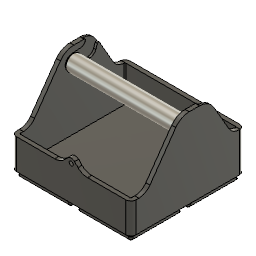
SnapTools-2U-Solder-Wire-Holder (Autodesk Fusion 360 design; units mm, degrees)
Autodesk Fusion 360 part; units mm, degrees
sketch "Sketch1" plane through (0, 0, 0) normal (0, 1, 0) x (1, 0, 0) in component "SnapTools-2U-Solder-Wire-Holder-Base"
  line L0 (-41.75, -2.4) -> (-2.4, -2.4)
  line L1 (-2.4, -2.4) -> (-2.4, -39.6)
  line L2 (-2.4, -39.6) -> (-41.75, -39.6)
  line L3 (-41.75, -39.6) -> (-41.75, -2.4)
  line L4 (-41.75, 2.4) -> (-2.4, 2.4)
  line L5 (-2.4, 2.4) -> (-2.4, 39.6)
  line L6 (-2.4, 39.6) -> (-41.75, 39.6)
  line L7 (-41.75, 39.6) -> (-41.75, 2.4)
  line L8 (-41.75, 2.4) -> (-2.4, 39.6) construction
  circle A0 centre (-35.8263, 8) radius 3.125
  line L9 (-22.075, 21) -> (-2.4, 21) construction
  line L10 (-2.4, 2.4) -> (-22.075, 21) construction
  circle A1 centre (-8.3237, 8) radius 3.125
  circle A2 centre (-8.3237, 34) radius 3.125
  circle A3 centre (-35.8263, 34) radius 3.125
  line L11 (0, 0) -> (34, 0) construction
  circle A4 centre (-35.8263, -34) radius 3.125
  circle A5 centre (-35.8263, -8) radius 3.125
  circle A6 centre (-8.3237, -8) radius 3.125
  circle A7 centre (-8.3237, -34) radius 3.125
  circle A8 centre (-22.075, 21) radius 5.125
  circle A9 centre (-22.075, -21) radius 5.125
  line L12 (0, 0) -> (0, 26) construction
  line L13 (2.4, 2.4) -> (2.4, 39.6)
  line L14 (41.75, 2.4) -> (2.4, 2.4)
  line L15 (41.75, 39.6) -> (41.75, 2.4)
  line L16 (2.4, 39.6) -> (41.75, 39.6)
  circle A10 centre (35.8263, 34) radius 3.125
  circle A11 centre (22.075, 21) radius 5.125
  circle A12 centre (8.3237, 34) radius 3.125
  circle A13 centre (8.3237, 8) radius 3.125
  circle A14 centre (35.8263, 8) radius 3.125
  circle A15 centre (35.8263, -8) radius 3.125
  circle A16 centre (8.3237, -8) radius 3.125
  line L17 (2.4, -39.6) -> (41.75, -39.6)
  line L18 (41.75, -39.6) -> (41.75, -2.4)
  line L19 (2.4, -2.4) -> (2.4, -39.6)
  line L20 (41.75, -2.4) -> (2.4, -2.4)
  circle A17 centre (22.075, -21) radius 5.125
  circle A18 centre (8.3237, -34) radius 3.125
  circle A19 centre (35.8263, -34) radius 3.125
  dimension "d15" = 39.35
  dimension "d16" = 4.8
  dimension "d18" = 2.4
  dimension "d19" = 79.2
  dimension "d20" = 39.6
  dimension "d21" = 37.2
  dimension "d25" = 5.6
  dimension "d26" = 6.25
  dimension "d27" = 6.25
  dimension "d28" = 5.6
  dimension "d110" = 10.25
  constraint horizontal L0
  constraint vertical L1
  constraint horizontal L2
  constraint vertical L3
  constraint horizontal L4
  constraint vertical L5
  constraint horizontal L6
  constraint vertical L7
  constraint collinear L1 L5
  constraint collinear L3 L7
  constraint coincident L8 A0.centre
  constraint midpoint L8 L9.start
  constraint midpoint L5 L9.end
  constraint coincident L10 A1.centre
  constraint symmetric A0 L9 A3
  constraint symmetric L9 A1 A2
  constraint coincident L11.start L12.start
  constraint parallel L4 L11
  constraint symmetric A0 L11 A5
  constraint symmetric A1 L11 A6
  constraint symmetric A2 L11 A7
  constraint symmetric A3 L11 A4
  constraint coincident L9.start L10.end
  constraint symmetric L11 A8 A9
  constraint perpendicular L11 L12
  constraint symmetric L0.start L12 L18.end
  constraint symmetric L0.end L12 L19.start
  constraint symmetric L1.end L12 L17.start
  constraint symmetric L2.end L12 L17.end
  constraint symmetric L4.start L12 L14.start
  constraint symmetric L4.end L12 L13.start
  constraint symmetric L5.end L12 L13.end
  constraint symmetric L6.end L12 L15.start
  constraint symmetric A0 L12 A14
  constraint symmetric A1 L12 A13
  constraint symmetric A2 L12 A12
  constraint symmetric A3 L12 A10
  constraint symmetric A4 L12 A19
  constraint symmetric A5 L12 A15
  constraint symmetric A6 L12 A16
  constraint symmetric A7 L12 A18
  constraint symmetric A8 L12 A11
  constraint symmetric A9 L12 A17
  measures "d15" distance of L1.end L2.end
  measures "d16" distance of L0 L4
  measures "d18" vertical distance of L11.start L0.end
  measures "d19" distance of L2 L6
  measures "d20" distance of L11.start L2
  measures "d21" distance of L0 L2
  measures "d25" distance of L4 A0.centre
  measures "d26" diameter of A0
  measures "d27" diameter of A1
  measures "d28" distance of L4 A1.centre
  measures "d74" angle of L4.start
  measures "d110" diameter of A8
extrude "Extrude1" add sketch "Sketch1" along normal blind 2.6 contours L0 L1 L2 L3 | L4 L5 L6 L7 | A0 | A1 | A2 | A3 | A4 | A5 | A6 | A7 | A8 | A9 | L13 L14 L15 L16 | A10 | A11 | A12 | A13 | A14 | A15 | A16 | L17 L18 L19 L20 | A17 | A18 | A19 makes body 1 at (-28.6333, 0, 27.2) makes body 2 at (-15.5167, 0, -27.2) makes body 3 at (15.5167, 0, 14.8) makes body 4 at (15.5167, 0, -27.2) in component "SnapTools-2U-Solder-Wire-Holder-Base"
fillet "Fillet3" radius 1.6 16 edges at (-2.4, 1.3, 2.4) (-41.75, 1.3, 2.4) (-41.75, 1.3, 39.6) (-2.4, 1.3, 39.6) (-41.75, 1.3, -39.6) (-41.75, 1.3, -2.4) (-2.4, 1.3, -2.4) (-2.4, 1.3, -39.6) (2.4, 1.3, 39.6) (2.4, 1.3, 2.4) (41.75, 1.3, 39.6) (41.75, 1.3, 2.4) (41.75, 1.3, -2.4) (2.4, 1.3, -2.4) (2.4, 1.3, -39.6) (41.75, 1.3, -39.6) on bodies 1 2 3 4 in component "SnapTools-2U-Solder-Wire-Holder-Base"
chamfer "Chamfer4" distance 0.8 angle 45 32 edges at (-41.75, 0, -21) (-41.2814, 0, -2.8686) (-22.075, 0, -2.4) (-2.8686, 0, -2.8686) (-2.4, 0, -21) (-2.8686, 0, -39.1314) (-22.075, 0, -39.6) (-41.2814, 0, -39.1314) (-41.75, 0, 21) (-41.2814, 0, 2.8686) (-22.075, 0, 2.4) (-2.8686, 0, 2.8686) (-2.4, 0, 21) (-2.8686, 0, 39.1314) (-22.075, 0, 39.6) (-41.2814, 0, 39.1314) (22.075, 0, 39.6) (41.2814, 0, 39.1314) (41.75, 0, 21) (41.2814, 0, 2.8686) (22.075, 0, 2.4) (2.8686, 0, 2.8686) (2.4, 0, 21) (2.8686, 0, 39.1314) (22.075, 0, -2.4) (2.8686, 0, -2.8686) (2.4, 0, -21) (2.8686, 0, -39.1314) (22.075, 0, -39.6) (41.2814, 0, -39.1314) (41.75, 0, -21) (41.2814, 0, -2.8686) on bodies 1 2 3 4 in component "SnapTools-2U-Solder-Wire-Holder-Base"
extrude "Extrude7" add 4 faces at (-16.05, 2.6, -27.2) (16.05, 2.6, -27.2) (16.05, 2.6, 14.8) (-28.1, 2.6, 27.2) along direction (0, 1, 0) blind 2.15 draft 45 on bodies 1 2 3 4 bodies 2 3 1 4 in component "SnapTools-2U-Solder-Wire-Holder-Base"
sketch "Sketch6" plane through (0, 4.75, 0) normal (0, 1, 0) x (-1, 0, 0) in component "SnapTools-2U-Solder-Wire-Holder-Base"
  line L0 (0.25, -4) -> (0.25, -38)
  arc A0 (0.25, -38) -> (4, -41.75) centre (4, -38) ccw
  line L1 (4, -41.75) -> (40.15, -41.75)
  arc A1 (40.15, -41.75) -> (43.9, -38) centre (40.15, -38) ccw
  line L2 (43.9, -38) -> (43.9, -4)
  arc A2 (43.9, -4) -> (40.15, -0.25) centre (40.15, -4) ccw
  line L3 (40.15, -0.25) -> (4, -0.25)
  arc A3 (4, -0.25) -> (0.25, -4) centre (4, -4) ccw
  line L4 (40.15, 41.75) -> (4, 41.75)
  arc A4 (4, 41.75) -> (0.25, 38) centre (4, 38) ccw
  line L5 (0.25, 38) -> (0.25, 4)
  arc A5 (0.25, 4) -> (4, 0.25) centre (4, 4) ccw
  line L6 (4, 0.25) -> (40.15, 0.25) construction
  arc A6 (40.15, 0.25) -> (43.9, 4) centre (40.15, 4) ccw
  line L7 (43.9, 4) -> (43.9, 38)
  arc A7 (43.9, 38) -> (40.15, 41.75) centre (40.15, 38) ccw
  line L8 (43.9, -4) -> (43.9, 4)
  line L9 (40.15, 41.75) -> (4, 41.75)
  arc A8 (4, 41.75) -> (0.25, 38) centre (4, 38) ccw
  line L10 (0.25, 38) -> (0.25, 4)
  arc A9 (0.25, 4) -> (4, 0.25) centre (4, 4) ccw
  line L11 (4, 0.25) -> (40.15, 0.25)
  arc A10 (40.15, 0.25) -> (43.9, 4) centre (40.15, 4) ccw
  line L12 (43.9, 4) -> (43.9, 38)
  arc A11 (43.9, 38) -> (40.15, 41.75) centre (40.15, 38) ccw
  line L13 (-43.9, 38) -> (-43.9, 4)
  arc A12 (-43.9, 4) -> (-40.15, 0.25) centre (-40.15, 4) ccw
  line L14 (-40.15, 0.25) -> (-4, 0.25)
  arc A13 (-4, 0.25) -> (-0.25, 4) centre (-4, 4) ccw
  line L15 (-0.25, 4) -> (-0.25, 38)
  arc A14 (-0.25, 38) -> (-4, 41.75) centre (-4, 38) ccw
  line L16 (-4, 41.75) -> (-40.15, 41.75)
  arc A15 (-40.15, 41.75) -> (-43.9, 38) centre (-40.15, 38) ccw
  line L17 (-43.9, -4) -> (-43.9, -38)
  arc A16 (-43.9, -38) -> (-40.15, -41.75) centre (-40.15, -38) ccw
  line L18 (-40.15, -41.75) -> (-4, -41.75)
  arc A17 (-4, -41.75) -> (-0.25, -38) centre (-4, -38) ccw
  line L19 (-0.25, -38) -> (-0.25, -4)
  arc A18 (-0.25, -4) -> (-4, -0.25) centre (-4, -4) ccw
  line L20 (-4, -0.25) -> (-40.15, -0.25)
  arc A19 (-40.15, -0.25) -> (-43.9, -4) centre (-40.15, -4) ccw
  line L21 (0.25, -4) -> (0.25, -38)
  arc A20 (0.25, -38) -> (4, -41.75) centre (4, -38) ccw
  line L22 (4, -41.75) -> (40.15, -41.75)
  arc A21 (40.15, -41.75) -> (43.9, -38) centre (40.15, -38) ccw
  line L23 (43.9, -38) -> (43.9, -4)
  arc A22 (43.9, -4) -> (40.15, -0.25) centre (40.15, -4) ccw
  line L24 (40.15, -0.25) -> (4, -0.25)
  arc A23 (4, -0.25) -> (0.25, -4) centre (4, -4) ccw
  line L25 (4, 41.75) -> (-4, 41.75)
  line L26 (-43.9, 4) -> (-43.9, -4)
  line L27 (-4, -41.75) -> (4, -41.75)
  constraint coincident L2.end A2.start
  constraint coincident A6.end L7.start
  constraint coincident L4.end A4.start
  constraint coincident A14.end L16.start
  constraint coincident L13.end A12.start
  constraint coincident L17.start A19.end
  constraint coincident L18.end A17.start
  constraint coincident A0.end L1.start
extrude "Extrude10" add sketch "Sketch6" along normal blind 2.25 bodies 1 3 4 2 in component "SnapTools-2U-Solder-Wire-Holder-Base"
extrude "Extrude5" cut sketch "Sketch1" along normal blind 2 contours A0 | A1 | A2 | A3 | A4 | A5 | A6 | A7 | A10 | A12 | A13 | A14 | A15 | A16 | A18 | A19 bodies 1 in component "SnapTools-2U-Solder-Wire-Holder-Base"
extrude "Extrude6" cut 16 faces at (-35.0627, 2, -35.019) (-7.3389, 2, -33.241) (-36.6468, 2, -8.8534) (-7.9632, 2, -7.548) (-7.4113, 2, 8.7544) (-36.8217, 2, 6.89) (-35.0627, 2, 32.981) (-7.3389, 2, 34.759) (9.0194, 2, 36.0626) (36.5899, 2, 32.981) (9.236, 2, 8.7544) (34.831, 2, 6.89) (34.831, 2, -9.11) (7.9948, 2, -9.1373) (8.9223, 2, -35.9409) (36.5899, 2, -35.019) along direction (0, 1, 0) blind 5 draft -55 on bodies 1 bodies 1 in component "SnapTools-2U-Solder-Wire-Holder-Base"
sketch "Sketch1 (2)" plane through (0, 7, 0) normal (0, 1, 0) x (-1, 0, 0) in component "SnapTools-2U-Solder-Wire-Holder-Base"
  line L0 (-40.15, -41.75) -> (40.15, -41.75)
  arc A0 (40.15, -41.75) -> (43.9, -38) centre (40.15, -38) ccw
  line L1 (43.9, -38) -> (43.9, 38)
  line L2 (31.464, -31.8398) -> (-31.536, -31.8398) construction
  line L3 (-31.536, -31.8398) -> (-31.536, 31.1602) construction
  line L4 (-31.536, 31.1602) -> (31.464, 31.1602) construction
  line L5 (31.464, 31.1602) -> (31.464, -31.8398) construction
  arc A1 (43.9, 38) -> (40.15, 41.75) centre (40.15, 38) ccw
  line L6 (40.15, 41.75) -> (-40.15, 41.75)
  arc A2 (-40.15, 41.75) -> (-43.9, 38) centre (-40.15, 38) ccw
  line L7 (-43.9, 38) -> (-43.9, -38)
  arc A3 (-43.9, -38) -> (-40.15, -41.75) centre (-40.15, -38) ccw
  line L8 (-40.15, -38.75) -> (40.15, -38.75)
  arc A4 (40.15, -38.75) -> (40.9, -38) centre (40.15, -38) ccw
  line L9 (40.9, -38) -> (40.9, 38)
  arc A5 (40.9, 38) -> (40.15, 38.75) centre (40.15, 38) ccw
  line L10 (40.15, 38.75) -> (-40.15, 38.75)
  arc A6 (-40.15, 38.75) -> (-40.9, 38) centre (-40.15, 38) ccw
  line L11 (-40.9, 38) -> (-40.9, -38)
  arc A7 (-40.9, -38) -> (-40.15, -38.75) centre (-40.15, -38) ccw
  dimension "d67" = 63
  dimension "d68" = 63
  constraint horizontal L2
  constraint vertical L3
  constraint horizontal L4
  constraint vertical L5
  measures "d67" distance of L2.start L2.end
  measures "d68" distance of L2.start L4.end
extrude "Extrude11" add sketch "Sketch1 (2)" along normal blind 56.5 bodies 1 in component "SnapTools-2U-Solder-Wire-Holder-Base"
sketch "Sketch2" plane through (-43.9, 0, 0) normal (-1, 0, 0) x (0, 0, 1) in component "SnapTools-2U-Solder-Wire-Holder-Base"
  line L0 (-38, 4.75) -> (-4, 4.75)
  line L1 (38, 63.5) -> (-38, 63.5)
  line L2 (-38, 63.5) -> (-38, 4.75)
  line L3 (-38, 7) -> (-38.75, 7)
  line L4 (-38, 7) -> (38, 7)
  circle A0 centre (0, 53.5) radius 5 construction
  circle A1 centre (0, 53.5) radius 31.5 construction
  line L5 (41.75, 4.75) -> (41.75, 63.5)
  line L6 (41.75, 27) -> (30.7632, 27)
  line L7 (30.7632, 27) -> (5.2057, 63.5)
  line L8 (-15.5885, 63.5) -> (-32.909, 33.5)
  line L9 (-41.75, 4.75) -> (-41.75, 63.5)
  line L10 (-32.909, 33.5) -> (-41.75, 33.5)
  line L11 (0, 7) -> (0, 63.5) construction
  line L12 (-15.5885, 63.5) -> (-41.75, 63.5)
  line L13 (5.2057, 63.5) -> (41.75, 63.5)
  line L14 (-4, 4.75) -> (4, 4.75)
  line L15 (4, 4.75) -> (38, 4.75)
  line L16 (38, 4.75) -> (38, 63.5)
  line L17 (38.75, 7) -> (38, 7)
  line L18 (38.75, 7) -> (38, 7)
  line L19 (38, 7) -> (-38, 7)
  line L20 (-38, 7) -> (-38.75, 7)
  dimension "d71" = 10
  dimension "d73" = 63
  dimension "d74" = 125
  dimension "d75" = 10
  dimension "d76" = 120
  dimension "d77" = 30
  dimension "d78" = 18.5
  dimension "d130" = 46.5
  dimension "d132" = 20
  constraint concentric A0 A1
  constraint coincident L5 L6.start
  constraint coincident L1 L7.end
  constraint coincident L1 L8.start
  constraint coincident L9 L10.end
  constraint perpendicular L9 L10
  constraint midpoint L1 L11.end
  constraint coincident A0.centre L11
  constraint coincident L9.end L12.end
  constraint coincident L5.end L13.end
  constraint midpoint L4 L11.start
  constraint perpendicular L5 L6
  measures "d71" diameter of A0
  measures "d73" diameter of A1
  measures "d74" angle of L6 L7
  measures "d75" distance of A0.centre L7
  measures "d76" angle of L8 L10
  measures "d77" distance of L1 L10
  measures "d78" distance of A0.centre L8
  measures "d130" distance of A0.centre L19
  measures "d132" distance of L4 L6
extrude "Extrude12" cut sketch "Sketch2" against normal through all contours L2 L9 L10 L12 | L1 L2 L8 L10 L12 | L5 L6 L13 L16 | L1 L6 L7 L13 L16 bodies 1 in component "SnapTools-2U-Solder-Wire-Holder-Base"
sketch "Sketch3" plane through (40.9, 0, 0) normal (-1, 0, 0) x (0, 0, 1) in component "SnapTools-2U-Solder-Wire-Holder-Base"
  line L0 (0, 0) -> (0, 69) construction
  circle A0 centre (0, 53.5) radius 5 construction
  circle A1 centre (0, 53.5) radius 5.25
  line L1 (0.4576, 58.73) -> (-6.6468, 59.3516)
  line L2 (-9.2044, 61.3141) -> (-10, 63.5)
  line L3 (-0.4576, 48.27) -> (-12.9564, 49.3635)
  line L4 (-17.2191, 52.6344) -> (-19.0142, 57.5664)
  arc A2 (-9.2044, 61.3141) -> (-6.6468, 59.3516) centre (-6.3853, 62.3402) ccw
  arc A3 (-17.2191, 52.6344) -> (-12.9564, 49.3635) centre (-12.5206, 54.3445) ccw
  line L5 (-32.909, 33.5) -> (-38, 33.5)
  line L6 (-38, 33.5) -> (-38, 7)
  line L7 (-38, 7) -> (38, 7)
  line L8 (38, 7) -> (38, 27)
  line L9 (38, 27) -> (30.7632, 27)
  line L10 (30.7632, 27) -> (5.2057, 63.5)
  line L11 (5.2057, 63.5) -> (-15.5885, 63.5)
  line L12 (-15.5885, 63.5) -> (-32.909, 33.5)
  dimension "d80" = 10
  dimension "d82" = 0.25
  dimension "d83" = 10.5
  dimension "d86" = 3
  dimension "d87" = 5
  dimension "d88" = 10
  dimension "d133" = 46.5
  dimension "d134" = 70
  dimension "d135" = 5
  constraint coincident L0 A0.centre
  constraint coincident A1 L1.start
  constraint coincident A1 L3.start
  constraint parallel L2 L4
  constraint tangent A1 L1
  constraint tangent A1 L3
  constraint parallel L1 L3
  constraint tangent L2 A2
  constraint tangent L1 A2
  constraint tangent L4 A3
  constraint tangent L3 A3
  constraint coincident L4.end L12
  constraint coincident L2.end L11
  constraint coincident L0.start origin
  constraint vertical L0
  measures "d80" diameter of A0
  measures "d83" distance of L2 L4
  measures "d86" radius of A2
  measures "d87" radius of A3
  measures "d88" horizontal distance of A0.centre L2.end
  measures "d133" distance of A0.centre L7
  measures "d134" angle of L2 L11
  measures "d135" angle of L1 L11
extrude "Extrude13" cut sketch "Sketch3" against normal blind 1.6 contours A1 | A1 L1 L2 L3 L4 A2 A3 L11 L12 bodies 1 in component "SnapTools-2U-Solder-Wire-Holder-Base"
extrude "Extrude14" cut 1 faces at (42.5, 52.3283, -6.6869) along direction (-1, 0, 0) blind 1.6 from surface at 83.4 on bodies 1 bodies 1 in component "SnapTools-2U-Solder-Wire-Holder-Base"
sketch "Sketch7" plane through (0, 0, 41.75) normal (0, 0, 1) x (1, 0, 0) in component "SnapTools-2U-Solder-Wire-Holder-Base"
  line L0 (40.15, 27) -> (-40.15, 27)
  line L1 (-40.15, 27) -> (-40.15, 4.75)
  circle A0 centre (0, 30) radius 1.5
  circle A1 centre (0, 30) radius 3.5
  line L2 (0, 27) -> (0, 36.6034) construction
  line L3 (-2.4749, 32.4749) -> (-7.9497, 27)
  line L4 (2.4749, 32.4749) -> (7.9497, 27)
  line L5 (-40.15, 4.75) -> (-4, 4.75)
  line L6 (-4, 4.75) -> (4, 4.75)
  line L7 (4, 4.75) -> (40.15, 4.75)
  line L8 (40.15, 4.75) -> (40.15, 27)
  dimension "d95" = 3
  dimension "d96" = 2
  dimension "d97" = 3
  dimension "d98" = 45
  dimension "d99" = 45
  constraint midpoint L0 L2.start
  constraint perpendicular L0 L2
  constraint coincident A0.centre L2
  constraint coincident A1 L3.start
  constraint coincident L0 L3.end
  constraint coincident A1 L4.start
  constraint coincident L0 L4.end
  constraint tangent A1 L4
  constraint tangent A1 L3
  measures "d95" diameter of A0
  measures "d97" distance of A0.centre L2.start
  measures "d98" angle of L0 L3
  measures "d99" angle of L0 L4
extrude "Extrude15" add sketch "Sketch7" against normal up to surface (3 mm away) contours L0 A1 L4 | L0 A1 | L0 A1 L3 picked at (-0.0374, 27.5014) bodies 1 in component "SnapTools-2U-Solder-Wire-Holder-Base"
fillet "Fillet4" radius 10 2 edges at (-7.9497, 27, 40.25) (7.9497, 27, 40.25) on bodies 1 in component "SnapTools-2U-Solder-Wire-Holder-Base"
fillet "Fillet5" radius 12 4 edges at (42.4, 63.5, 5.2057) (-42.4, 63.5, 5.2057) (-43.2, 63.5, -15.5885) (43.2, 63.5, -15.5885) on bodies 1 in component "SnapTools-2U-Solder-Wire-Holder-Base"
fillet "Fillet7" radius 10 4 edges at (-42.4, 27, 30.7632) (42.4, 27, 30.7632) (42.4, 33.5, -32.909) (-42.4, 33.5, -32.909) on bodies 1 in component "SnapTools-2U-Solder-Wire-Holder-Base"
fillet "Fillet6" radius 0.8 4 edges at (-41.7, 57.5661, -19.0141) (41.7, 57.5661, -19.0141) (41.7, 63.4279, -9.9738) (-41.7, 63.4279, -9.9738) on bodies 1 in component "SnapTools-2U-Solder-Wire-Holder-Base"
extrude "Extrude16" cut sketch "Sketch1" along normal blind 5.25 contours A8 | A9 | A11 | A17 bodies 1 in component "SnapTools-2U-Solder-Wire-Holder-Base"
extrude "Extrude17" cut 4 faces at (-20.7203, 5.25, -21.7134) (-20.7203, 5.25, 20.2866) (23.4297, 5.25, -21.7134) (23.4297, 5.25, 20.2866) along direction (0, 1, 0) blind 0.8 draft -60 on bodies 1 bodies 1 in component "SnapTools-2U-Solder-Wire-Holder-Base"
sketch "Sketch1 (3)" plane through (42.5, 0, 0) normal (-1, 0, 0) x (0, 0, 1) in component "SnapTools-2U-Solder-Wire-Holder-Axle 10mm"
  line L0 (-18.4274, 55.9543) -> (-17.2191, 52.6344)
  arc A0 (-17.2191, 52.6344) -> (-12.9564, 49.3635) centre (-12.5206, 54.3445) ccw
  line L1 (-12.9564, 49.3635) -> (-0.4576, 48.27)
  line L2 (0.4576, 58.73) -> (-6.6468, 59.3516)
  arc A1 (-9.2044, 61.3141) -> (-6.6468, 59.3516) centre (-6.3853, 62.3402) ccw
  circle A2 centre (0, 53.5) radius 5
  line L3 (-9.2044, 61.3141) -> (-9.6086, 62.4247)
  arc A3 (-8.8709, 63.4982) -> (-19.0526, 57.5) centre (-8.6603, 51.5) ccw
  line L4 (-19.0526, 57.5) -> (-19.872, 56.0807)
  arc A4 (-18.4274, 55.9543) -> (-19.872, 56.0807) centre (-19.1792, 55.6807) ccw
  arc A5 (-0.4576, 48.27) -> (0.4576, 58.73) centre (0, 53.5) ccw
  arc A6 (-8.8709, 63.4982) -> (-9.6086, 62.4247) centre (-8.8569, 62.6983) ccw
  dimension "d115" = 10
  constraint coincident A2.centre A5.centre
  measures "d115" diameter of A2
extrude "Extrude1'" add sketch "Sketch1 (3)" along normal up to surface (85 mm away) separate body contours A2 makes body 5 in component "SnapTools-2U-Solder-Wire-Holder-Axle 10mm"
sketch "Sketch1 (4)" plane through (42.5, 0, 0) normal (-1, 0, 0) x (0, 0, 1) in component "SnapTools-2U-Solder-Wire-Holder-Axle 20mm"
  line L0 (-18.4274, 55.9543) -> (-17.2191, 52.6344)
  arc A0 (-17.2191, 52.6344) -> (-12.9564, 49.3635) centre (-12.5206, 54.3445) ccw
  line L1 (-12.9564, 49.3635) -> (-0.4576, 48.27)
  line L2 (0.4576, 58.73) -> (-6.6468, 59.3516)
  arc A1 (-9.2044, 61.3141) -> (-6.6468, 59.3516) centre (-6.3853, 62.3402) ccw
  circle A2 centre (0, 53.5) radius 5
  circle A3 centre (0, 53.5) radius 10
  line L3 (-9.2044, 61.3141) -> (-9.6086, 62.4247)
  arc A4 (-8.8709, 63.4982) -> (-19.0526, 57.5) centre (-8.6603, 51.5) ccw
  line L4 (-19.0526, 57.5) -> (-19.872, 56.0807)
  arc A5 (-18.4274, 55.9543) -> (-19.872, 56.0807) centre (-19.1792, 55.6807) ccw
  arc A6 (-0.4576, 48.27) -> (0.4576, 58.73) centre (0, 53.5) ccw
  arc A7 (-8.8709, 63.4982) -> (-9.6086, 62.4247) centre (-8.8569, 62.6983) ccw
  dimension "d115_1" = 10
  dimension "d119" = 20
  constraint concentric A2 A3
  constraint coincident A2.centre A3.centre
  measures "d115_1" diameter of A2
  measures "d119" diameter of A3
extrude "Extrude1''" add sketch "Sketch1 (4)" along normal up to surface (85 mm away) separate body contours A2 makes body 6 in component "SnapTools-2U-Solder-Wire-Holder-Axle 20mm"
extrude "Extrude2" add sketch "Sketch1 (4)" along normal up to surface (81.3 mm away) from surface at 1.85 contours L1 L2 A1 A3 A6 | L1 L2 A1 A3 A6 bodies 6 in component "SnapTools-2U-Solder-Wire-Holder-Axle 20mm"
chamfer "Chamfer1" distance 5 angle 45 2 edges at (-40.65, 49.8838, -9.3233) (40.65, 57.1162, -9.3233) on bodies 6 in component "SnapTools-2U-Solder-Wire-Holder-Axle 20mm"
sketch "Sketch1 (5)" plane through (42.5, 0, 0) normal (-1, 0, 0) x (0, 0, 1) in component "SnapTools-2U-Solder-Wire-Holder-Axle Parametric"
  line L0 (-18.4274, 55.9543) -> (-17.2191, 52.6344)
  arc A0 (-17.2191, 52.6344) -> (-12.9564, 49.3635) centre (-12.5206, 54.3445) ccw
  line L1 (-12.9564, 49.3635) -> (-0.4576, 48.27)
  line L2 (0.4576, 58.73) -> (-6.6468, 59.3516)
  arc A1 (-9.2044, 61.3141) -> (-6.6468, 59.3516) centre (-6.3853, 62.3402) ccw
  circle A2 centre (0, 53.5) radius 5
  circle A3 centre (0, 53.5) radius 5.75
  line L3 (-9.2044, 61.3141) -> (-9.6086, 62.4247)
  arc A4 (-8.8709, 63.4982) -> (-19.0526, 57.5) centre (-8.6603, 51.5) ccw
  line L4 (-19.0526, 57.5) -> (-19.872, 56.0807)
  arc A5 (-18.4274, 55.9543) -> (-19.872, 56.0807) centre (-19.1792, 55.6807) ccw
  arc A6 (-0.4576, 48.27) -> (0.4576, 58.73) centre (0, 53.5) ccw
  arc A7 (-8.8709, 63.4982) -> (-9.6086, 62.4247) centre (-8.8569, 62.6983) ccw
  dimension "d115_1_1" = 10
  dimension "d119_1" = 11.5
  constraint concentric A2 A3
  constraint coincident A2.centre A3.centre
  measures "d115_1_1" diameter of A2
  measures "d119_1" diameter of A3
extrude "Extrude1'''" add sketch "Sketch1 (5)" along normal up to surface (85 mm away) separate body contours A2 makes body 7 in component "SnapTools-2U-Solder-Wire-Holder-Axle Parametric"
extrude "Extrude2'" add sketch "Sketch1 (5)" along normal up to surface (81.3 mm away) from surface at 1.85 contours L1 L2 A3 A6 | L1 L2 A3 A6 bodies 7 in component "SnapTools-2U-Solder-Wire-Holder-Axle Parametric"
chamfer "Chamfer1'" distance 0.75 angle 45 2 edges at (-40.65, 51.4207, -5.3609) (40.65, 55.5793, -5.3609) on bodies 7 in component "SnapTools-2U-Solder-Wire-Holder-Axle Parametric"
sketch "Sketch4" plane through (40.9, 0, 0) normal (-1, 0, 0) x (0, 0, 1)
  arc A0 (-18.6485, 57) -> (-27.841, 52.7135) centre (-18.6485, 45) ccw
  line L0 (-27.841, 52.7135) -> (-29.0383, 51.2865)
  arc A1 (-36.4, 47.1405) -> (-29.0383, 51.2865) centre (-38.2309, 59) ccw
  line L1 (-36.4, 47.1405) -> (-36.4, 4.75)
  line L2 (-36.4, 4.75) -> (-5.6, 4.75)
  line L3 (-5.6, 4.75) -> (5.6, 4.75)
  line L4 (5.6, 4.75) -> (36.4, 4.75)
  line L5 (36.4, 4.75) -> (36.4, 22.8096)
  arc A2 (30.0399, 26.7571) -> (36.4, 22.8096) centre (39.2324, 34.4706) ccw
  line L6 (30.0399, 26.7571) -> (8.2599, 52.7135)
  arc A3 (8.2599, 52.7135) -> (-0.9326, 57) centre (-0.9326, 45) ccw
  line L7 (-0.9326, 57) -> (-18.6485, 57)
  circle A4 centre (-0.3007, 53.6477) radius 25
  circle A5 centre (-0.3007, 53.6477) radius 5
  line L8 (-4, 4.75) -> (-38, 4.75)
  line L9 (-38, 4.75) -> (-38, 42.0565)
  arc A6 (-20.7187, 55.7495) -> (-24.5775, 52.7135) centre (-15.385, 45) ccw
  line L10 (-20.7187, 55.7495) -> (-17.2191, 46.1344)
  arc A7 (-17.2191, 46.1344) -> (-12.9564, 42.8635) centre (-12.5207, 47.8445) ccw
  line L11 (-12.9564, 42.8635) -> (-4, 42.0799)
  line L12 (-4, 42.0799) -> (-4, 4.75)
  arc A8 (-38, 42.0565) -> (-29.9703, 46.2865) centre (-39.1629, 54) ccw
  line L13 (-29.9703, 46.2865) -> (-24.5775, 52.7135)
  arc A9 (-8.8709, 63.4982) -> (-9.6086, 62.4247) centre (-8.8569, 62.6983) ccw
  line L14 (-9.6086, 62.4247) -> (-9.2044, 61.3141)
  arc A10 (-9.2044, 61.3141) -> (-6.6468, 59.3516) centre (-6.3853, 62.3402) ccw
  line L15 (-6.6468, 59.3516) -> (0.4576, 58.73)
  arc A11 (-0.4576, 48.27) -> (0.4576, 58.73) centre (0, 53.5) ccw
  line L16 (-0.4576, 48.27) -> (-12.9564, 49.3635)
  arc A12 (-17.2191, 52.6344) -> (-12.9564, 49.3635) centre (-12.5206, 54.3445) ccw
  line L17 (-17.2191, 52.6344) -> (-18.4274, 55.9543)
  arc A13 (-18.4274, 55.9543) -> (-19.872, 56.0807) centre (-19.1792, 55.6807) ccw
  line L18 (-19.872, 56.0807) -> (-30.0222, 38.5)
  line L19 (-38, 33.5233) -> (-38, 7)
  line L20 (-38, 7) -> (38, 7)
  line L21 (38, 7) -> (38, 27)
  line L22 (27.7774, 31.2642) -> (8.7887, 58.3829)
  arc A14 (8.7887, 58.3829) -> (-1.0411, 63.5) centre (-1.0411, 51.5) ccw
  line L23 (-1.0411, 63.5) -> (-8.6603, 63.5)
  arc A15 (-8.6603, 63.5) -> (-8.8709, 63.4982) centre (-8.6603, 51.5) ccw
  line L24 (38, 27) -> (35.9689, 27)
  arc A16 (-38, 33.5233) -> (-30.0222, 38.5) centre (-38.6825, 43.5) ccw
  arc A17 (27.7774, 31.2642) -> (35.9689, 27) centre (35.9689, 37) ccw
  dimension "d125" = 50
  dimension "d126" = 10
  constraint concentric A4 A5
  measures "d125" diameter of A4
  measures "d126" diameter of A5
component "SnapTools-2U-Solder-Wire-Holder-Base" placed x (1, 0, 0) y (0, 1, 0) z (0, 0, 1) at (0, 0, 0)
component "SnapTools-2U-Solder-Wire-Holder-Axle 10mm" placed x (1, 0, 0) y (0, 1, 0) z (0, 0, 1) at (0, 0, 0)
component "SnapTools-2U-Solder-Wire-Holder-Axle 20mm" placed x (1, 0, 0) y (0, 1, 0) z (0, 0, 1) at (0, 0, 0)
component "SnapTools-2U-Solder-Wire-Holder-Axle Parametric" placed x (1, 0, 0) y (0, 1, 0) z (0, 0, 1) at (0, 0, 0)
equation "printer_offset = 0.25 mm"
equation "solder_spool_width = 63 mm"
equation "solder_spool_diameter = 63 mm"
equation "solder_spool_center_hole_diameter = 11.5 mm"
equation "holder_axle_diameter = 10 mm"
equation "holder_width = 41.5 mm" comment "gridfinity width"
equation "holder_length = 83.5 mm"
equation "holder_solder_spool_bottom_spacing = 15 mm"
equation "holder_axle_slot_angle = 5 deg"
equation "holder_axle_depth = 10 mm"
equation "gridfinity_bottom_chamfer = 0.8 mm"
equation "gridfinity_top_chamfer = 2.15 mm"
equation "gridfinity_chamfer_offset = 0.25 mm"
equation "gridfinity_chamfer_spacing = 1.8 mm"
equation "d15 = holder_width - gridfinity_top_chamfer"
equation "d16 = 2 * ( gridfinity_top_chamfer + gridfinity_chamfer_offset )"
equation "d18 = d16 / 2"
equation "d19 = holder_length - ( 2 * gridfinity_top_chamfer )"
equation "d20 = d19 / 2"
equation "gridfinity_magnet_hole_size = 6 mm"
equation "gridfinity_magnet_hole_depth = 2 mm"
equation "gridfinity_distance_from_side = gridfinity_bottom_chamfer + 4.8 mm"
equation "d25 = gridfinity_distance_from_side"
equation "d26 = gridfinity_magnet_hole_size + printer_offset"
equation "d27 = d26"
equation "d28 = d25"
equation "d29 = gridfinity_bottom_chamfer + gridfinity_chamfer_spacing"
equation "gridfinity_1u = 7 mm"
equation "d44 = gridfinity_magnet_hole_depth"
equation "gridfinity_top_fillet_diameter = 7.5 mm"
equation "gridfinity_bottom_fillet_diameter = 3.2 mm"
equation "d54 = gridfinity_top_chamfer"
equation "d61 = gridfinity_bottom_fillet_diameter / 2"
equation "d62 = gridfinity_bottom_chamfer"
equation "d63 = gridfinity_1u - gridfinity_bottom_chamfer - gridfinity_chamfer_spacing - gridfinity_top_chamfer"
equation "d67 = solder_spool_width"
equation "d68 = solder_spool_diameter"
equation "d69 = solder_spool_diameter / 2 + holder_solder_spool_bottom_spacing + holder_axle_depth"
equation "d71 = holder_axle_diameter"
equation "d73 = solder_spool_diameter"
equation "d80 = holder_axle_diameter"
equation "d82 = printer_offset"
equation "d83 = holder_axle_diameter + 2 * printer_offset"
equation "d87 = holder_axle_diameter / 2"
equation "holder_axle_slot_length = 10 mm"
equation "snaptool_magnet_diameter = 10 mm"
equation "snaptool_magnet_depth = 5 mm"
equation "d110 = snaptool_magnet_diameter + printer_offset"
equation "d111 = snaptool_magnet_depth + printer_offset"
equation "d115 = holder_axle_diameter"
equation "d115_1 = holder_axle_diameter"
equation "d120 = printer_offset"
equation "d121 = printer_offset"
equation "d115_1_1 = holder_axle_diameter"
equation "d119_1 = holder_axle_parametric_size"
equation "d120_1 = printer_offset"
equation "d121_1 = printer_offset"
equation "d123_1 = ( holder_axle_parametric_size - holder_axle_diameter ) / 2"
equation "holder_axle_parametric_size = 11.5 mm"
equation "d127 = ( gridfinity_top_chamfer + gridfinity_chamfer_offset )"
equation "d128 = -wall_thickness"
equation "wall_thickness = 3 mm"
equation "d130 = solder_spool_diameter / 2 + holder_solder_spool_bottom_spacing"
equation "d133 = solder_spool_diameter / 2 + holder_solder_spool_bottom_spacing"
named bodies: "SnapTools-2U-Solder-Wire-Holder-Base", "SnapTools-2U-Solder-Wire-Holder-Axle 10mm", "SnapTools-2U-Solder-Wire-Holder-Axle 20mm", "SnapTools-2U-Solder-Wire-Holder-Axle Parametric"
